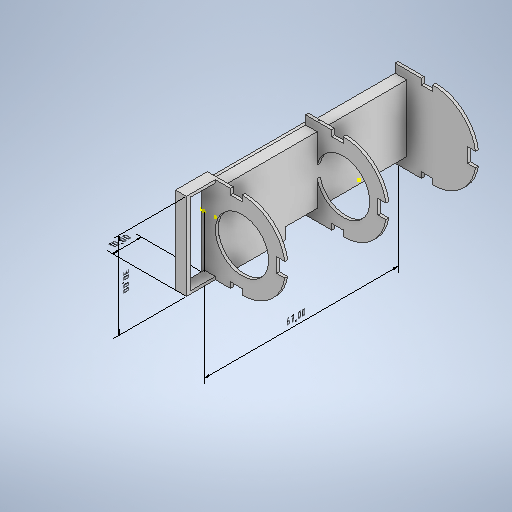
# Autodesk Inventor part: Part4
Saved by Autodesk Inventor 2025.3 (Build 293356000, 356)
## iProperties
Created: 2025-06-07
Part Number: Part4
Material: Generic
Document SubType Name: Modeling
Designer: Repete
Density: 1 g/cm^3
Appearance: Default
Author: Repete
Autodesk Inventor part; units mm, degrees
sketch "Sketch1" plane through (0, 0, 0) normal (0, 1, 0) x (-1, 0, 0)
  circle A0 centre (4.631591, -3.797233) radius 9.2
  line L0 (17.631591, 11.202767) -> (4.631591, 11.202767)
  line L1 (4.631591, -18.797233) -> (17.631591, -18.797233)
  line L2 (17.631591, -18.797233) -> (17.631591, 11.202767)
  arc A1 (4.631591, 11.202767) -> (-10.158608, -1.297233) centre (4.631591, -3.797233) ccw
  arc A2 (-10.158608, -6.297233) -> (4.631591, -18.797233) centre (4.631591, -3.797233) ccw
  arc A3 (-10.158608, -1.297233) -> (-10.158608, -6.297233) centre (4.631591, -3.797233) ccw
  point P0 (17.631591, -3.797233)
  dimension "d6" = 30
  dimension "d7" = 18.4
  dimension "d13" = 13
  constraints: 6 end point, 6 point on circle, 4 centre point, 2 concentric, 1 coincident, 1 horizontal, 1 midpoint, 1 parallel
  measures "d6" distance of L1.end L0.start
  measures "d7" diameter of A0
  measures "d13" distance of point (17.632, -3.797) A0.centre
extrude "Extrusion1" add sketch "Sketch1" along normal blind 1
sketch "Sketch5" plane through (0, 1, 0) normal (0, 1, 0) x (1, 0, 0)
  line L0 (-17.631591, 18.797233) -> (-17.631591, -11.202767)
  line L1 (-4.631591, 18.797233) -> (-17.631591, 18.797233)
  line L2 (-17.631591, -11.202767) -> (-13.631591, -11.202767)
  line L3 (-13.631591, -11.202767) -> (-13.631591, 18.797233)
  line L4 (-13.631591, 18.797233) -> (-17.631591, 18.797233)
  line L5 (-17.631591, 18.797233) -> (-17.631591, -11.202767)
  point P0 (0, 0)
  dimension "d17" = 4
  constraints: 8 end point, 2 parallel, 1 horizontal, 1 perpendicular, 1 point on line
  measures "d17" distance between parallel lines of L0 L3
extrude "Extrusion2" add sketch "Sketch5" along normal blind 35
sketch "Sketch6" plane through (-17.631591, 0, -18.797233) normal (-1, 0, 0) x (0, 0, 1)
  line L0 (0, 0) -> (0, 36) projected
  line L1 (0, 1) -> (25, 1)
  line L2 (25, 1) -> (25, 35)
  line L3 (25, 35) -> (0, 35)
  line L4 (0, 35) -> (0, 1)
  line L5 (0, 0) -> (30, 0) projected
  point P0 (18.797233, 0)
  point P1 (0, 35)
  point P2 (0, 35)
  dimension "d20" = 25
  dimension "d21" = 1
  dimension "d22" = 34
  constraints: 8 end point, 2 parallel, 1 horizontal, 1 perpendicular, 1 point on line
  measures "d20" distance of L1.start L1.end
  measures "d21" distance between parallel lines of L5 L1
  measures "d22" distance between parallel lines of L1 L3
extrude "Extrusion3" cut sketch "Sketch6" against normal blind 3
sketch "Sketch7" plane through (-17.631591, 0, -18.797233) normal (-1, 0, 0) x (0, 0, 1)
  point P0 (18.797233, 0)
sketch "Sketch8" plane through (-17.631591, 0, -18.797233) normal (-1, 0, 0) x (0, 0, 1)
  line L0 (30, 1) -> (30, 36) projected
  line L1 (25, 35) -> (25, 1) projected
  line L2 (30, 15) -> (25, 15)
  line L3 (25, 15) -> (25, 23)
  line L4 (25, 23) -> (30, 23)
  line L5 (30, 23) -> (30, 15)
  line L6 (0, 0) -> (30, 0) projected
  point P0 (18.797233, 0)
  point P1 (27.5, 15)
  point P2 (27.5, 23)
  point P3 (24, 34.5)
  dimension "d27" = 15
  dimension "d28" = 8
  constraints: 8 end point, 2 midpoint, 2 parallel, 1 horizontal, 1 perpendicular, 1 point on line, 2 other
  measures "d27" distance from line of L6 point (27.5, 15)
  measures "d28" distance of point (27.5, 15) point (27.5, 23)
extrude "Extrusion4" [suppressed]
sketch "Sketch9" plane through (-14.631591, 35, 6.202767) normal (0, 0, -1) x (-1, 0, 0)
  line L0 (3, -12) -> (3.5, -12) projected
  line L1 (3, 0) -> (3, -34) projected
  line L2 (3.5, -12) -> (3, -12)
  line L3 (3, -12) -> (3, -20)
  line L4 (3, -20) -> (3.5, -20)
  line L5 (3.5, -20) -> (3.5, -12)
  point P0 (-14.631591, -35)
  constraints: 8 end point, 2 parallel, 1 horizontal, 1 perpendicular
extrude "Extrusion5" [suppressed]
sketch "Sketch12" plane through (-18.131591, 23, 11.202767) normal (0, 1, 0) x (1, 0, 0)
  line L0 (0, 0) -> (0, 22)
  line L1 (0.5, 5) -> (0.5, 22)
  line L2 (0, 22) -> (0.5, 22)
  line L3 (0.5, 15.461966) -> (0, 15.461966)
  line L4 (0, 15.461966) -> (0, 22)
  line L5 (0.5, 15.461966) -> (1.933369, 18.768927)
  line L6 (1.933369, 18.768927) -> (1.933369, 22)
  line L7 (1.933369, 22) -> (0.5, 22)
  point P0 (18.131591, 11.202767)
  dimension "d36" = 0.5
  constraints: 12 end point, 1 horizontal, 1 parallel, 1 perpendicular, 1 point on line, 1 vertical
  measures "d36" distance of L0.end L2.end
extrude "Extrusion6" [suppressed]
fillet "Fillet1" [suppressed]
sketch "Sketch20" plane through (0, 36, 0) normal (0, 1, 0) x (1, 0, 0)
  point P0 (0, 0)
ref_plane "Work Plane1" through (0, 36, 0) normal (0, -1, 0) x (1, 0, 0)
sketch "Sketch24" plane through (-4.631591, 0, -18.797233) normal (0, 0, -1) x (-1, 0, 0)
  line L0 (0, 0) -> (-14.790199, 0)
  line L1 (0, 1) -> (9, 1)
  line L2 (0, 0) -> (4, 0)
  line L3 (4, 0) -> (4, 1)
  line L4 (4, 1) -> (0, 1)
  line L5 (0, 1) -> (0, 0)
  point P0 (-4.631591, 0)
  dimension "d69" = 4
  constraints: 8 end point, 2 parallel, 1 horizontal, 1 perpendicular, 1 point on line
  measures "d69" distance between parallel lines of L3 L5
extrude "Extrusion16" cut sketch "Sketch24" against normal blind 2
sketch "Sketch25" plane through (-17.631591, 0, 11.202767) normal (0, 0, 1) x (1, 0, 0)
  line L0 (4, 1) -> (13, 1) projected
  line L1 (3.8, 0) -> (22.2, 0) projected
  line L2 (13, 1) -> (9, 1)
  line L3 (9, 1) -> (9, 0)
  line L4 (9, 0) -> (13, 0)
  line L5 (13, 0) -> (13, 1)
  point P0 (17.631591, 0)
  dimension "d72" = 4
  constraints: 8 end point, 2 parallel, 1 horizontal, 1 perpendicular, 1 point on line
  measures "d72" distance between parallel lines of L3 L5
extrude "Extrusion17" cut sketch "Sketch25" against normal blind 2
sketch "Sketch30" plane through (-13.631591, 1, -1.889355) normal (1, 0, 0) x (0, 0, -1)
  point P0 (-1.889355, -1)
sketch "Sketch31" plane through (-13.631591, 1, -1.889355) normal (1, 0, 0) x (0, 0, -1)
  line L0 (-13.092122, 0) -> (-13.092122, 35)
  line L1 (16.907878, 0) -> (-13.092122, 0)
  line L2 (-13.092122, 34) -> (-10.092122, 34)
  line L3 (-10.092122, 34) -> (-10.092122, 0)
  line L4 (-10.092122, 0) -> (-13.092122, 0)
  line L5 (-13.092122, 0) -> (-13.092122, 34)
  line L6 (-13.092122, 35) -> (16.907878, 35)
  point P0 (-1.889355, -1)
  point P1 (-11.592122, 34)
  dimension "d97" = 3
  dimension "d100" = 1
  constraints: 8 end point, 2 parallel, 2 point on line, 1 horizontal, 1 midpoint, 1 perpendicular
  measures "d97" distance of L2.start L2.end
  measures "d100" distance from line of L6 point (-11.592, 34)
extrude "Extrusion22" cut sketch "Sketch31" against normal through all
sketch "Sketch32" plane through (0, 36, 0) normal (0, -1, 0) x (1, 0, 0)
  circle A0 centre (-4.655217, -3.803606) radius 9.2
  line L0 (-17.655217, -18.803606) -> (-8.631591, -18.803606)
  line L1 (-8.631591, 11.196394) -> (-17.655217, 11.196394)
  line L2 (-17.655217, 11.196394) -> (-17.655217, -18.803606)
  arc A1 (-4.655217, -18.803606) -> (10.134983, -6.303606) centre (-4.655217, -3.803606) ccw
  arc A2 (10.134983, -6.303606) -> (-4.655217, 11.196394) centre (-4.655217, -3.803606) ccw
  line L3 (-4.631591, 9.202767) -> (-4.631591, 11.202767)
  line L4 (-4.631591, 9.202767) -> (-8.631591, 9.202767)
  line L5 (-8.631591, 9.202767) -> (-8.631591, 11.196394)
  line L6 (-4.631591, 11.196375) -> (-4.631591, 9.202767)
  line L7 (-4.631591, -16.797233) -> (-8.631591, -16.797233)
  line L8 (-8.631591, -16.797233) -> (-4.631591, -16.797233)
  line L9 (-4.631591, -16.797233) -> (-4.631591, -18.803588)
  line L10 (-8.631591, -18.803606) -> (-8.631591, -16.797233)
  arc A3 (10.134983, -6.303606) -> (10.134983, -6.303606) centre (-3.06837, -4.071832) ccw
  point P0 (0, 0)
  point P1 (-17.655217, -3.803606)
  point P2 (-4.631591, -16.797233)
  point P3 (10.134983, -6.303606)
  dimension "d101" = 30
  dimension "d102" = 18.4
  dimension "d103" = 13
  constraints: 18 end point, 8 point on circle, 4 centre point, 3 parallel, 2 horizontal, 2 perpendicular, 1 coincident, 1 midpoint, 1 tangent
  measures "d101" distance of L1.end L0.start
  measures "d102" diameter of A0
  measures "d103" distance of point (-17.655, -3.804) A0.centre
sketch "Sketch32 outline for Extrusion23" plane through (0, 36, 0) normal (0, -1, 0) x (1, 0, 0)
  line L0 (-8.631591, -18.803606) -> (-8.631591, -16.797233)
  line L1 (-17.655217, -18.803606) -> (-8.631591, -18.803606)
  line L2 (-8.631591, -16.797233) -> (-4.631591, -16.797233)
  line L3 (-17.655217, 11.196394) -> (-17.655217, -18.803606)
  line L4 (-4.631591, -16.797233) -> (-4.631591, -18.803588)
  line L5 (-8.631591, 11.196394) -> (-17.655217, 11.196394)
  arc A0 (-4.631591, -18.803588) -> (10.134983, -6.303606) centre (-4.655217, -3.803606) ccw
  line L6 (-8.631591, 9.202767) -> (-8.631591, 11.196394)
  arc A1 (10.134983, -6.303606) -> (-4.631591, 11.196375) centre (-4.655217, -3.803606) ccw
  line L7 (-4.631591, 9.202767) -> (-8.631591, 9.202767)
  line L8 (-4.631591, 11.196375) -> (-4.631591, 9.202767)
  circle A2 centre (-4.655217, -3.803606) radius 9.2
extrude "Extrusion23" add sketch "Sketch32 outline for Extrusion23" along normal blind 1
ref_plane "Work Plane3" through (0, 66, 0) normal (0, 1, 0) x (1, 0, 0)
sketch "Sketch34" plane through (0, 66, 0) normal (0, 1, 0) x (1, 0, 0)
  line L0 (-17.655217, -11.199121) -> (-8.631591, -11.199121)
  line L1 (-8.631591, 18.800879) -> (-17.655217, 18.800879)
  line L2 (-17.655217, 18.800879) -> (-17.655217, -11.199121)
  arc A0 (-4.655217, -11.199121) -> (10.134983, 1.300879) centre (-4.655217, 3.800879) ccw
  arc A1 (10.134983, 6.300879) -> (-4.655217, 18.800879) centre (-4.655217, 3.800879) ccw
  line L3 (-4.631591, 16.800879) -> (-8.631591, 16.800879)
  line L4 (-8.631591, 16.800879) -> (-8.631591, 18.800879)
  line L5 (-4.631591, 18.80086) -> (-4.631591, 16.800879)
  line L6 (-8.631591, -9.199121) -> (-4.631591, -9.199121)
  line L7 (-4.631591, -9.199121) -> (-4.631591, -11.199103)
  line L8 (-8.631591, -11.199121) -> (-8.631591, -9.199121)
  arc A2 (10.134983, 1.300879) -> (10.134983, 6.300879) centre (-4.655217, 3.800879) ccw
  point P0 (0, 0)
  point P1 (-17.655217, 3.800879)
  dimension "d113" = 30
  dimension "d137" = 2
  dimension "d138" = 2
  constraints: 18 end point, 8 point on circle, 3 centre point, 3 parallel, 2 horizontal, 2 perpendicular, 1 midpoint
  measures "d113" distance of L1.end L0.start
  measures "d137" distance between parallel lines of L6 L0
  measures "d138" distance between parallel lines of L1 L3
extrude "Extrusion25" add sketch "Sketch34" along normal blind 1
sketch "Sketch13" plane through (-14.631591, 0, -18.797233) normal (-1, 0, 0) x (0, 0, 1)
  line L0 (0, 35) -> (25, 35) projected
  line L1 (0, 35) -> (4, 35)
  line L2 (4, 35) -> (4, 24)
  line L3 (4, 24) -> (0, 24)
  line L4 (0, 24) -> (0, 35)
  point P0 (18.797233, 0)
  dimension "d37" = 11
  dimension "d38" = 4
  constraints: 8 end point, 2 parallel, 1 horizontal, 1 perpendicular
  measures "d37" distance of L3.end L0.start
  measures "d38" distance of L2.end L3.end
extrude "Extrusion7" cut sketch "Sketch13" along normal through all both and the other way through all
sketch "Sketch33" plane through (0, 36, 0) normal (0, 1, 0) x (1, 0, 0)
  line L0 (-17.631591, -8.202767) -> (-13.631591, -8.202767)
  line L1 (-13.631591, -8.202767) -> (-13.631591, 14.797233)
  line L2 (-13.631591, 14.797233) -> (-14.631591, 14.797233)
  line L3 (-17.631591, -6.202767) -> (-17.631591, -8.202767)
  line L4 (-17.631591, 18.797233) -> (-17.631591, -11.202767)
  line L5 (-17.631591, -6.202767) -> (-14.631591, -6.202767)
  line L6 (-14.631591, -6.202767) -> (-14.631591, 14.797233)
  point P0 (0, 0)
  constraints: 12 end point, 2 horizontal, 2 parallel, 2 perpendicular, 2 other
extrude "Extrusion24" add sketch "Sketch33" along normal up to surface (30 mm away)
sketch "Sketch35" plane through (0, 0, 0) normal (0, -1, 0) x (1, 0, 0)
  line L0 (-17.631591, 11.202767) -> (-8.631591, 11.202767)
  line L1 (-17.631591, -18.797233) -> (-14.631591, -18.797233)
  line L2 (-13.86512, 11.202767) -> (-17.631591, 11.202767)
  line L3 (-17.631591, 11.202767) -> (-17.631591, -18.797233)
  line L4 (-17.631591, -18.797233) -> (-13.86512, -18.797233)
  line L5 (-13.86512, -18.797233) -> (-13.86512, 11.202767)
  point P0 (0, 0)
  constraints: 8 end point, 2 parallel, 1 horizontal, 1 perpendicular, 1 point on line
extrude "Extrusion26" add sketch "Sketch35" along normal blind 10
sketch "Sketch36" plane through (-13.86512, 0, 11.202767) normal (1, 0, 0) x (0, 0, -1)
  line L0 (0, 0) -> (30, 0) projected
  line L1 (1, 0) -> (29, 0)
  line L2 (29, 0) -> (29, -8.5)
  line L3 (29, -8.5) -> (1, -8.5)
  line L4 (1, -8.5) -> (1, 0)
  line L5 (30, 0) -> (30, -10) projected
  line L6 (0, 0) -> (0, -10) projected
  line L7 (30, -10) -> (0, -10) projected
  point P0 (11.202767, 0)
  point P1 (29, 0)
  dimension "d126" = 1
  dimension "d127" = 1
  dimension "d128" = 1.5
  constraints: 8 end point, 2 parallel, 1 horizontal, 1 perpendicular, 1 point on line
  measures "d126" distance between parallel lines of L5 L2
  measures "d127" distance between parallel lines of L6 L4
  measures "d128" distance between parallel lines of L7 L3
extrude "Extrusion27" cut sketch "Sketch36" against normal through all contours L0 L2 L3 L4
sketch "Sketch37" plane through (0, 67, 0) normal (0, 1, 0) x (1, 0, 0)
  line L0 (12.349926, 1.300879) -> (7.344783, 1.300879)
  line L1 (7.344783, 1.300879) -> (7.344783, 6.300879)
  line L2 (7.344783, 6.300879) -> (12.349926, 6.300879)
  line L3 (12.349926, 6.300879) -> (12.349926, 1.300879)
  arc A0 (-4.631591, -11.199103) -> (-4.631591, 18.80086) centre (-4.655217, 3.800879) ccw
  line L4 (-4.631591, 16.800879) -> (-8.631591, 16.800879)
  point P0 (0, 0)
  point P1 (12.349926, 3.800879)
  point P2 (9.847354, 1.300879)
  point P3 (9.847354, 6.300879)
  dimension "d140" = 5
  dimension "d143" = 10.5
  dimension "d146" = 12
  constraints: 8 end point, 3 midpoint, 2 parallel, 1 horizontal, 1 perpendicular
  measures "d140" distance between parallel lines of L2 L0
  measures "d143" distance from line of point (9.847, 6.301) L4
  measures "d146" distance from line of A0.centre L1
extrude "Extrusion28" cut sketch "Sketch37" against normal through all
ref_plane "Work Plane4" through (-18.631591, 1, 6.202767) normal (-1, 0, 0) x (0, 0, 1)
sketch "Sketch38" plane through (-18.631591, 1, 6.202767) normal (-1, 0, 0) x (0, 0, 1)
  line L0 (5, -1) -> (-7.503645, -1)
  line L1 (-25.006373, 35) -> (1.993627, 35)
  line L2 (1.993627, 35) -> (1.993627, -1)
  line L3 (1.993627, -1) -> (-25.006373, -1)
  line L4 (-25.006373, -1) -> (-25.006373, 35)
  point P0 (-6.202767, -1)
  constraints: 8 end point, 2 parallel, 1 horizontal, 1 perpendicular, 1 point on line
extrude "Extrusion29" add sketch "Sketch38" against normal up to surface (1 mm away)
sketch "Sketch39" plane through (-18.631591, 1, 6.202767) normal (-1, 0, 0) x (0, 0, 1)
  point P0 (-6.202767, -1)
sketch "Sketch40" plane through (-18.631591, 1, 6.202767) normal (-1, 0, 0) x (0, 0, 1)
  line L0 (-25.006373, 34) -> (-21.006373, 34)
  line L1 (-21.006373, 34) -> (-21.006373, 23)
  line L2 (-21.006373, 23) -> (-25.006373, 23)
  line L3 (-25.006373, 23) -> (-25.006373, 34)
  line L4 (-25.006373, 35) -> (-25.006373, -1)
  point P0 (-6.202767, -1)
  dimension "d150" = 4
  dimension "d153" = 0
  constraints: 8 end point, 2 parallel, 1 horizontal, 1 perpendicular
  measures "d150" distance of L1.end L2.end
  measures "d153" distance between parallel lines of L4 L3
extrude "Extrusion30" cut sketch "Sketch40" against normal blind 10
sketch "Sketch41" plane through (-18.631591, 1, 6.202767) normal (-1, 0, 0) x (0, 0, 1)
  line L0 (-4.006373, 5) -> (-28.006373, 5)
  line L1 (-28.006373, 5) -> (-28.006373, 30)
  line L2 (-28.006373, 30) -> (-4.006373, 30)
  line L3 (-4.006373, 30) -> (-4.006373, 5)
  line L4 (1.993627, -1) -> (1.993627, 35)
  line L5 (1.993627, 35) -> (-25.006373, 35)
  line L6 (-25.006373, -1) -> (1.993627, -1)
  point P0 (-6.202767, -1)
  dimension "d154" = 24
  dimension "d155" = 6
  dimension "d156" = 5
  dimension "d157" = 6
  constraints: 8 end point, 2 parallel, 1 horizontal, 1 perpendicular
  measures "d154" distance of L1.end L2.end
  measures "d155" distance between parallel lines of L4 L3
  measures "d156" distance between parallel lines of L5 L2
  measures "d157" distance between parallel lines of L6 L0
extrude "Extrusion31" cut sketch "Sketch41" against normal up to surface (1 mm away)
equation "\"d15\" = d45"
equation "\"d45\" = 1"
body "Solid1"
